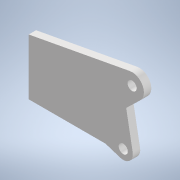
# Autodesk Inventor part: Metacarpo
Saved by Autodesk Inventor 2020 (Build 240168000, 168)
## iProperties
Created: 2021-08-13
Part Number: Metacarpo
Material: Generic
Document SubType Name: Modeling
Designer: chalo
Density: 1 g/cm^3
Appearance: Default
Author: chalo
Autodesk Inventor part; units mm, degrees
ref_plane "YZ Plane" through (0, 0, 0) normal (1, 0, 0) x (0, 1, 0)
ref_plane "XZ Plane" through (0, 0, 0) normal (0, 1, 0) x (-1, 0, 0)
ref_plane "XY Plane" through (0, 0, 0) normal (0, 0, 1) x (1, 0, 0)
sketch "Sketch1" plane through (0, 0, 0) normal (0, 0, 1) x (1, 0, 0)
  circle A0 centre (-3.75, 4.5) radius 1.55 projected
  circle A1 centre (-3.75, 4.5) radius 3.25
  line L0 (-0.5539, 5.0893) -> (-2.75, 17)
  line L1 (-2.75, 17) -> (0.6336, 22.3667)
  circle A2 centre (-2.75, 24.5) radius 4
  circle A3 centre (-2.75, 24.5) radius 1.55
  line L2 (-4.75, 1.4077) -> (-9.75, 3.0246)
  line L3 (-9.75, 3.0246) -> (-35.75, 3.0246)
  line L4 (-35.75, 3.0246) -> (-35.75, 22.0246)
  line L5 (-4.154, 28.2455) -> (-20.75, 22.0246)
  line L6 (-20.75, 22.0246) -> (-35.75, 22.0246)
  point P0 (0, 0)
  dimension "d0" = 6.5
  dimension "d2" = 8
  dimension "d4" = 1
  dimension "d5" = 1
  dimension "d6" = 3.1
  dimension "d7" = 20
  dimension "d8" = 12.5
  dimension "d9" = 26
  dimension "d10" = 5
  dimension "d11" = 32
  dimension "d12" = 19
  dimension "d15" = 15
  constraints: 14 end point, 4 point on circle, 4 tangent, 3 centre point, 2 coincident, 1 horizontal, 1 perpendicular, 1 vertical
  measures "d0" diameter of A1
  measures "d2" diameter of A2
  measures "d4" horizontal distance of A2.centre A0.centre
  measures "d5" horizontal distance of A0.centre L0.end
  measures "d6" diameter of A3
  measures "d7" vertical distance of A0.centre A2.centre
  measures "d8" vertical distance of A0.centre L0.end
  measures "d9" distance of L2.end L3.end
  measures "d10" horizontal distance of L2.start L2.end
  measures "d11" horizontal distance of L3.end A0.centre
  measures "d12" distance of L3.end L4.end
  measures "d15" distance of L5.end L4.end
ref_plane "Work Plane1" through (0, -6.7, 2.5) normal (0, 0, 1) x (1, 0, 0)
extrude "Extrusion1" add sketch "Sketch1" along normal up to surface (2.5 mm away)
ref_plane "Work Plane2" through (21.6, 23.8, -5.75) normal (0, 0, 1) x (1, 0, 0)
mirror "Mirror1" about plane through (21.6, 23.8, -5.75) normal (0, 0, 1) of "Extrusion1"
body "Solid1"
